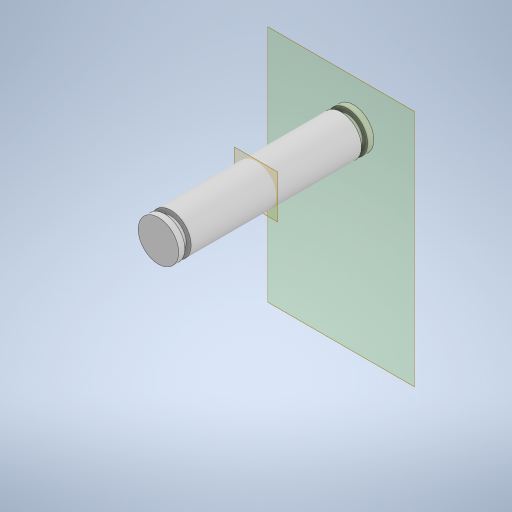
# Autodesk Inventor part: axle
Saved by Autodesk Inventor 2024 (Build 280153000, 153)
## iProperties
Created: 2024-03-08
Part Number: axle
Material: Generic
Document SubType Name: Modeling
Designer: MaartenGeorgesBuelen
Density: 1 g/cm^3
Appearance: Default
Sheet Metal Rule: Default
Author: MaartenGeorgesBuelen
## iProperties of the stored document axle_3DPrint.ipt
Created: 2024-03-08
Part Number: axle_3DPrint
Material: Generic
Document SubType Name: Modeling
Designer: MaartenGeorgesBuelen
Density: 1 g/cm^3
Appearance: Default
Author: MaartenGeorgesBuelen
Autodesk Inventor part; units mm, degrees
ref_plane "YZ Plane" through (0, 0, 0) normal (1, 0, 0) x (0, 1, 0)
ref_plane "XZ Plane" through (0, 0, 0) normal (0, 1, 0) x (-1, 0, 0)
ref_plane "Work Plane1" through (70, 0, -110) normal (0, 0, -1) x (-1, 0, 0)
sketch "Sketch1" plane through (70, 0, -110) normal (0, 0, -1) x (-1, 0, 0)
  circle A0 centre (35, 110) radius 13.5 projected
  circle A1 centre (35, 110) radius 13.09
  point P0 (70, 0)
  dimension "d2" = 0.41
  constraints: 1 centre point
  measures "d2" radial gap between concentric circles of A0 A1
ref_plane "Work Plane2" through (-8, 0, 0) normal (0, 0, 1) x (1, 0, 0)
extrude "Extrusion1" add sketch "Sketch1" against normal up to surface (110 mm away) contours A1
sketch "Sketch2" plane through (35, 110, 0) normal (0, 0, 1) x (1, 0, 0)
  circle A0 centre (0, 0) radius 13.09 projected
  circle A1 centre (0, 0) radius 10
  point P0 (-35, -110)
  dimension "d3" = 20
  constraints: 1 centre point, 1 coincident
  measures "d3" diameter of A1
extrude "Extrusion2" add sketch "Sketch2" along normal blind 4 contours A1
sketch "Sketch3" plane through (35, 110, 4) normal (0, 0, 1) x (1, 0, 0)
  circle A0 centre (0, 0) radius 13.09 projected
  point P0 (-35, -110)
extrude "Extrusion3" add sketch "Sketch3" along normal blind 4
ref_plane "Work Plane3" through (35, 110, -55) normal (0, 0, 1) x (1, 0, 0)
mirror "Mirror1" about plane through (35, 110, -55) normal (0, 0, 1) of "Extrusion2", "Extrusion3"
equation "\"BendRadius\" = Thickness"
equation "\"BendReliefWidth\" = Thickness"
equation "\"BendReliefDepth\" = 0.5 * Thickness"
equation "\"CornerReliefSize\" = 4 * Thickness"
equation "\"MinimumRemnant\" = 2 * Thickness"
equation "\"TransitionRadius\" = BendRadius"
equation "\"JacobiRadiusSize\" = BendRadius"
equation "\"GapSize\" = Thickness"
equation "\"Thickness\" = 3.048"
body "Solid1"
